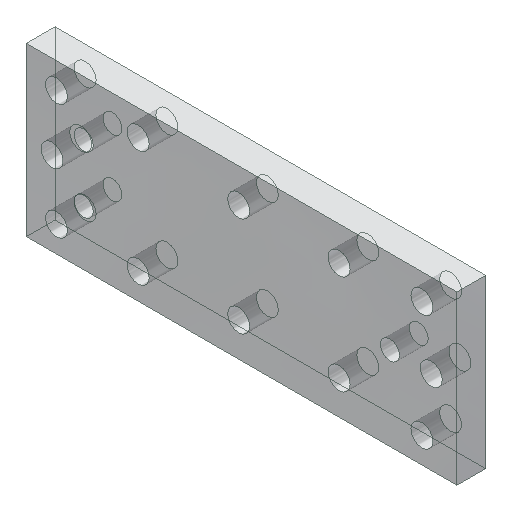
# Autodesk Inventor part: acrilico frontal
Saved by Autodesk Inventor 2025 (Build 290162000, 162)
## iProperties
Created: 2024-12-11
Part Number: acrilico frontal
Material: Acrílico, transparente
Document SubType Name: Modeling
Designer: November
Density: 1.19 g/cm^3
Appearance: Transparente
Author: November
Autodesk Inventor part; units mm, degrees
ref_plane "YZ Plane" through (0, 0, 0) normal (1, 0, 0) x (0, 1, 0)
ref_plane "XZ Plane" through (0, 0, 0) normal (0, 1, 0) x (-1, 0, 0)
ref_plane "XY Plane" through (0, 0, 0) normal (0, 0, 1) x (1, 0, 0)
sketch "Esboço1" plane through (0, 0, 0) normal (0, 0, 1) x (1, 0, 0)
  line L0 (90, 0) -> (0, 0)
  line L1 (0, 0) -> (0, -35)
  line L2 (0, -35) -> (90, -35)
  line L3 (90, -35) -> (90, 0)
  circle A0 centre (65.3687, -7.1) radius 2.3
  circle A1 centre (23.3687, -29.5996) radius 2.3
  circle A2 centre (44.3687, -27.9) radius 2.3
  circle A3 centre (44.3687, -7.1) radius 2.3
  circle A4 centre (84.63, -17.5) radius 2.3
  circle A5 centre (5.3687, -17.5) radius 2.3
  circle A6 centre (65.3687, -27.9) radius 2.3
  circle A7 centre (23.3687, -5.4004) radius 2.3
  circle A8 centre (12, -11.5) radius 2
  circle A9 centre (12, -23.5) radius 2
  circle A10 centre (76, -17.5) radius 2
  circle A11 centre (6.2932, -5.4004) radius 2.3
  circle A12 centre (6.2932, -29.5996) radius 2.3
  circle A13 centre (82.6841, -5.4004) radius 2.3
  circle A14 centre (82.6768, -29.5996) radius 2.3
  constraints: 15 centre point, 8 end point
extrude "Extrusão1" add sketch "Esboço1" along normal blind 6
